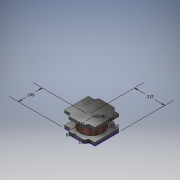
# Autodesk Inventor part: inductor
Saved by Autodesk Inventor 2019.3 (Build 233278000, 278)
## iProperties
Created: 2019-11-25
Part Number: inductor
Material: Generic
Document SubType Name: Modeling
Designer: kjdix
Density: 1 g/cm^3
Appearance: Steel Galvanized
Author: kjdix
Autodesk Inventor part; units mm, degrees
ref_plane "YZ Plane" through (0, 0, 0) normal (1, 0, 0) x (0, 1, 0)
ref_plane "XZ Plane" through (0, 0, 0) normal (0, 1, 0) x (-1, 0, 0)
ref_plane "XY Plane" through (0, 0, 0) normal (0, 0, 1) x (1, 0, 0)
sketch "Sketch1" plane through (0, 0, 0) normal (0, 1, 0) x (-1, 0, 0)
  line L0 (-4, 3.15) -> (4, 3.15)
  line L1 (4, 3.15) -> (4, -3.15)
  line L2 (4, -3.15) -> (-4, -3.15)
  line L3 (-4, -3.15) -> (-4, 3.15)
  line L4 (-4, 3.15) -> (4, -3.15) construction
  line L5 (4, 3.15) -> (-4, -3.15) construction
  line L6 (-2, 4) -> (2, 4)
  line L7 (2, 4) -> (2, -4)
  line L8 (2, -4) -> (-2, -4)
  line L9 (-2, -4) -> (-2, 4)
  line L10 (-2, 4) -> (2, -4) construction
  line L11 (2, 4) -> (-2, -4) construction
  line L12 (2, -4) -> (2.4907, -3.15)
  line L13 (2, -4) -> (2.9815, -4) construction
  line L14 (-2, -4) -> (-2.4907, -3.15)
  line L15 (-2, -4) -> (-1.0185, -4) construction
  line L16 (-2, 4) -> (-2.4907, 3.15)
  line L17 (-2, 4) -> (-1.0185, 4) construction
  line L18 (2, 4) -> (2.4907, 3.15)
  line L19 (2, 4) -> (2.9815, 4) construction
  point P0 (0, 0)
  dimension "d0" = 8
  dimension "d1" = 6.3
  dimension "d2" = 4
  dimension "d3" = 8
  dimension "d4" = 60
  dimension "d5" = 120
  dimension "d6" = 120
  dimension "d7" = 60
  constraints: 40 end point, 6 horizontal, 4 equal length, 4 midpoint, 4 parallel, 4 point on line, 2 perpendicular
  measures "d0" distance of L1.end L2.end
  measures "d1" distance of L0.end L1.end
  measures "d2" distance of L7.end L8.end
  measures "d3" distance of L6.end L7.end
  measures "d4" angle of L13 L12
  measures "d5" angle of L15 L14
  measures "d6" angle of L16 L17
  measures "d7" angle of L18 L19
extrude "Extrusion1" add sketch "Sketch1" along normal blind 4.2
extrude "Extrusion2" cut sketch "Sketch1" along normal blind 3.5
extrude "Extrusion3" add sketch "Sketch1" along normal blind 0.8
sketch "Sketch2" plane through (0, 0.8, 0) normal (0, 1, 0) x (1, 0, 0)
  circle A0 centre (0, 0) radius 3
  dimension "d14" = 6
  constraints: 1 centre point, 1 coincident
  measures "d14" diameter of A0
extrude "Extrusion4" add sketch "Sketch2" along normal up to next
body "Solid1"
